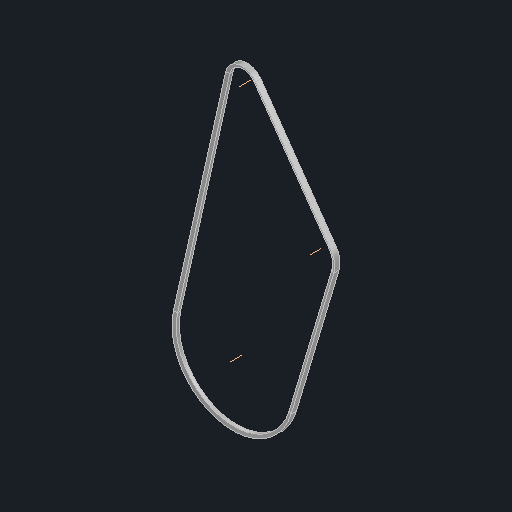
# Autodesk Inventor part: Courroie trapézoïdale
Saved by Autodesk Inventor 2026.2 (Build 302298010, 298A)
## iProperties
CustomPartVersion: 1
Created: 2026-03-31
Part Number: Courroie trapézoïdale
Material: Rubber
Document SubType Name: Modeling
Designer: romai
Density: 0.93 g/cm^3
Appearance: Rubber - Black - Version 1.1
Author: romai
Autodesk Inventor part; units mm, degrees
ref_plane "YZ Plane" through (0, 0, 0) normal (1, 0, 0) x (0, 1, 0)
ref_plane "XZ Plane" through (0, 0, 0) normal (0, 1, 0) x (-1, 0, 0)
sketch "Chemin d'esquisse" plane through (0, 0, 0) normal (0, 0, 1) x (1, 0, 0)
  arc A0 (-111.7313, 25.0274) -> (109.7586, -32.6082) centre (0, 0) ccw
  arc A1 (41.6622, 483.9245) -> (-11.2867, 473.4481) centre (17.5, 467) ccw
  arc A2 (191.7306, 243.3084) -> (186.1492, 277.6484) centre (153.387, 254.6999) ccw
  line L0 (191.7306, 243.3084) -> (109.7586, -32.6082)
  line L1 (-111.7313, 25.0274) -> (-11.2867, 473.4481)
  line L2 (41.6622, 483.9245) -> (186.1492, 277.6484)
  constraints: 6 end point, 6 point on circle, 3 centre point
ref_plane "Plan de section" through (109.7586, -32.6082, 0) normal (0.2848, 0.9586, 0) x (0, 0, 1)
sketch "Section" plane through (109.7586, -32.6082, 0) normal (0.2848, 0.9586, 0) x (0, 0, 1)
  line L0 (0, 2.4986) -> (0, -3.5014) construction
  line L1 (-4.25, 0) -> (4.25, 0) construction
  line L2 (-5.1594, 2.4986) -> (5.1594, 2.4986)
  line L3 (5.1594, 2.4986) -> (2.9756, -3.5014)
  line L4 (2.9756, -3.5014) -> (-2.9756, -3.5014)
  line L5 (-2.9756, -3.5014) -> (-5.1594, 2.4986)
  point P0 (0, 0)
  point P1 (0, 0)
  point P2 (0, 0)
  dimension "d0" = 8.5
  dimension "d1" = 2.4986
  dimension "d2" = 40
  dimension "d3" = 6
  constraints: 12 end point, 3 midpoint, 2 parallel, 2 point on line, 1 coincident, 1 perpendicular, 1 vertical, 1 other
  measures "d0" distance of L1.start L1.end
  measures "d1" distance between parallel lines of L2 L1
  measures "d2" angle of L5 L3
  measures "d3" distance between parallel lines of L4 L2
sweep "Courroie" add profiles "Section" path "Chemin d'esquisse"
equation "\"d0\" = da_Bw"
equation "\"d1\" = da_Hw"
equation "\"d2\" = da_Alfa"
equation "\"d3\" = da_H"
equation "\"da_Alfa\" = 40deg"
equation "\"da_H\" = 6"
equation "\"da_Bw\" = 8.5"
equation "\"da_Hw\" = 2.49859"
body "Solid1"
